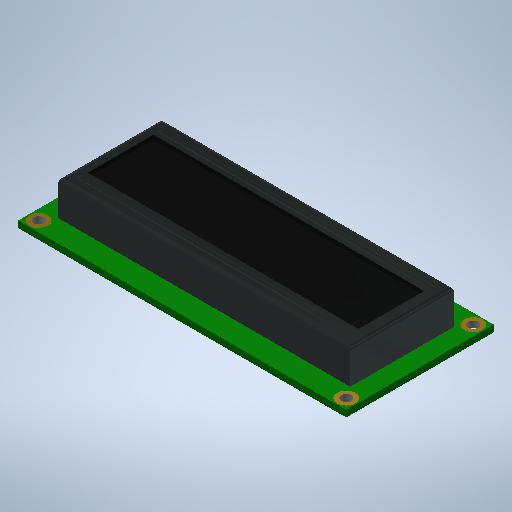
# Autodesk Inventor part: LCD
Saved by Autodesk Inventor 2025.3 (Build 293356000, 356)
## iProperties
Created: 2013-05-07
Part Number: LCD
Material: Generic
Document SubType Name: Modeling
Designer: Erika
Density: 1 g/cm^3
Appearance: Default
Author: Erika
Autodesk Inventor part; units mm, degrees
ref_plane "YZ Plane" through (0, 0, 0) normal (1, 0, 0) x (0, 1, 0)
ref_plane "XZ Plane" through (0, 0, 0) normal (0, 1, 0) x (-1, 0, 0)
ref_plane "XY Plane" through (0, 0, 0) normal (0, 0, 1) x (1, 0, 0)
sketch "Sketch1" plane through (0, 0, 0) normal (0, 0, 1) x (1, 0, 0)
  line L0 (-40, 18) -> (40, 18)
  line L1 (40, 18) -> (40, -18)
  line L2 (40, -18) -> (-40, -18)
  line L3 (-40, -18) -> (-40, 18)
  line L4 (-40, 18) -> (40, -18) construction
  line L5 (40, 18) -> (-40, -18) construction
  point P0 (0, 0)
  dimension "d0" = 80
  dimension "d2" = 36
  constraints: 12 end point, 2 midpoint, 2 parallel, 1 horizontal, 1 perpendicular
  measures "d0" distance of L0.start L0.end
  measures "d2" distance of L0.end L1.end
extrude "Extrusion1" add sketch "Sketch1" along normal blind 1.6
sketch "Sketch2" plane through (0, 0, 1.6) normal (0, 0, 1) x (1, 0, 0)
  line L0 (40, 18) -> (-40, 18) projected
  line L1 (-40, 18) -> (-40, -18) projected
  line L2 (-40, -18) -> (40, -18) projected
  line L3 (40, -18) -> (40, 18) projected
  circle A0 centre (-37.5, 15.5) radius 1.25
  circle A1 centre (37.5, 15.5) radius 1.25
  circle A2 centre (-37.5, -15.5) radius 1.25
  circle A3 centre (37.5, -15.5) radius 1.25
  line L4 (-50.5505, 0) -> (52.4138, 0)
  line L5 (0, 22.5117) -> (0, -22.0219)
  point P0 (0, 0)
  dimension "d5" = 2.5
  dimension "d6" = 2.5
  dimension "d7" = 2.5
  dimension "d8" = 2.5
  dimension "d9" = 75
  constraints: 4 centre point, 4 end point, 3 equal radius, 3 symmetric about line, 2 perpendicular
  measures "d5" distance from line of L1 A0.centre
  measures "d6" diameter of A0
  measures "d7" distance from line of L0 A1.centre
  measures "d8" distance from line of L2 A2.centre
  measures "d9" distance of A3.centre A2.centre
hole "Hole1" at (-37.5, 15.5, 1.6) at (-37.5, -15.5, 1.6) at (37.5, 15.5, 1.6) at (37.5, -15.5, 1.6) direction (0, 0, -1) diameter 2.5 depth 8 tip angle 118
sketch "Sketch3" plane through (0, 0, 1.6) normal (0, 0, 1) x (1, 0, 0)
  line L0 (-35.6, 12.6) -> (35.6, 12.6)
  line L1 (35.6, 12.6) -> (35.6, -12.6)
  line L2 (35.6, -12.6) -> (-35.6, -12.6)
  line L3 (-35.6, -12.6) -> (-35.6, 12.6)
  line L4 (-35.6, 12.6) -> (35.6, -12.6) construction
  line L5 (35.6, 12.6) -> (-35.6, -12.6) construction
  point P0 (0, 0)
  dimension "d17" = 25.2
  dimension "d19" = 71.2
  constraints: 12 end point, 2 midpoint, 2 parallel, 1 horizontal, 1 perpendicular
  measures "d17" distance of L2.end L0.start
  measures "d19" distance of L1.end L2.end
extrude "Extrusion2" add sketch "Sketch3" along normal blind 8.6
sketch "Sketch4" plane through (0, 0, 10.2) normal (0, 0, 1) x (1, 0, 0)
  line L0 (-33, 8) -> (33, 8)
  line L1 (33, 8) -> (33, -8)
  line L2 (33, -8) -> (-33, -8)
  line L3 (-33, -8) -> (-33, 8)
  line L4 (-33, 8) -> (33, -8) construction
  line L5 (33, 8) -> (-33, -8) construction
  point P0 (0, 0)
  dimension "d22" = 66
  dimension "d24" = 16
  constraints: 12 end point, 2 midpoint, 2 parallel, 1 horizontal, 1 perpendicular
  measures "d22" distance of L0.start L0.end
  measures "d24" distance of L0.end L1.end
extrude "Extrusion3" cut sketch "Sketch4" against normal blind 1
fillet "Fillet1" radius 1 4 edges at (0, -12.6, 10.2) (0, 12.6, 10.2) (-35.6, 0, 10.2) (35.6, 0, 10.2)
sketch "Sketch5" plane through (0, 0, 10.2) normal (0, 0, 1) x (1, 0, 0)
  line L0 (-34.6, 11.6) -> (34.6, 11.6) projected
  line L1 (-34.6, -11.6) -> (-34.6, 11.6) projected
  line L2 (34.6, -11.6) -> (-34.6, -11.6) projected
  line L3 (34.6, 11.6) -> (34.6, -11.6) projected
  line L4 (-33, 10.1) -> (33, 10.1)
  line L5 (33, 10.1) -> (33, 9.5)
  line L6 (33, 9.5) -> (-33, 9.5)
  line L7 (-33, 9.5) -> (-33, 10.1)
  line L8 (-33, -9.5) -> (32.1521, -9.5)
  line L9 (32.1521, -9.5) -> (32.1521, -10.1)
  line L10 (32.1521, -10.1) -> (-33, -10.1)
  line L11 (-33, -10.1) -> (-33, -9.5)
  point P0 (0, 0)
  dimension "d28" = 0.6
  dimension "d30" = 1.5
  dimension "d31" = 1.6
  dimension "d32" = 1.6
  dimension "d33" = 1.5
  dimension "d34" = 0.6
  constraints: 16 end point, 4 parallel, 2 horizontal, 2 perpendicular
  measures "d28" distance of L4.end L5.end
  measures "d30" distance between parallel lines of L0 L4
  measures "d31" distance between parallel lines of L1 L7
  measures "d32" distance between parallel lines of L3 L5
  measures "d33" distance between parallel lines of L2 L10
  measures "d34" distance of L8.end L9.end
extrude "Extrusion4" cut sketch "Sketch5" against normal blind 0.1 contours L4 L5 L6 L7 | L8 L9 L10 L11
fillet "Fillet2" radius 1 8 edges at (-0.4239, -10.1, 10.2) (-0.4239, -9.5, 10.2) (0, 9.5, 10.2) (0, 10.1, 10.2) (33, 9.8, 10.2) (-33, 9.8, 10.2) (-33, -9.8, 10.2) (32.1521, -9.8, 10.2)
sketch "Sketch8" plane through (0, 0, 1.6) normal (0, 0, 1) x (1, 0, 0)
  line L0 (40, 18) -> (-40, 18) projected
  line L1 (-40, 18) -> (-40, -18) projected
  line L2 (-31.1, 15.5) -> (-32.9, 15.5)
  line L3 (-32.9, 15.5) -> (-32.9, 18)
  line L4 (-32.9, 18) -> (-31.1, 18)
  line L5 (-31.1, 18) -> (-31.1, 15.5)
  line L6 (-31.1, 15.5) -> (-32.9, 18) construction
  line L7 (-32.9, 15.5) -> (-31.1, 18) construction
  circle A0 centre (-32, 15.5) radius 0.9
  point P0 (0, 0)
  point P1 (-32, 16.75)
  dimension "d56" = 1.8
  dimension "d58" = 2.5
  dimension "d59" = 8
  constraints: 12 end point, 3 midpoint, 2 parallel, 1 horizontal, 1 horizontal alignment, 1 perpendicular, 1 point on line, 2 other
  measures "d56" distance of L2.start L2.end
  measures "d58" distance between parallel lines of L0 L2
  measures "d59" distance from line of point (-32, 16.75) L1
extrude "Extrusion5" add sketch "Sketch8" along normal blind 0.01
pattern_linear "Rectangular Pattern1" count 16 spacing 2.54 along (1, 0, 0) of "Extrusion5"
sketch "Sketch10" plane through (0, 0, 1.61) normal (0, 0, 1) x (1, 0, 0)
  arc A0 (-32.9, 15.5) -> (-31.1, 15.5) centre (-32, 15.5) ccw projected
  circle A1 centre (-32, 15.5) radius 0.5
  point P0 (0, 0)
  dimension "d74" = 1
  constraints: 1 centre point, 1 coincident
  measures "d74" diameter of A1
hole "Hole4" at (-32, 15.5, 1.61) direction (0, 0, -1) diameter 1 end through all
pattern_linear "Rectangular Pattern2" count 16 spacing 2.54 along (1, 0, 0) of "Hole4"
sketch "Sketch11" plane through (0, 0, 1.6) normal (0, 0, 1) x (1, 0, 0)
  circle A0 centre (-37.5, 15.5) radius 1.25 projected
  circle A1 centre (-37.5, 15.5) radius 2.25
  point P0 (0, 0)
  dimension "d86" = 4.5
  constraints: 1 centre point, 1 coincident
  measures "d86" diameter of A1
extrude "Extrusion6" add sketch "Sketch11" along normal blind 0.01
pattern_linear "Rectangular Pattern3" count 2 spacing 31 along (0, -1, 0) count 2 spacing 75 along (1, 0, 0) of "Extrusion6"
body "Solid1"
